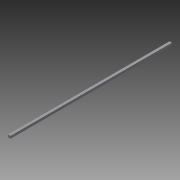
# Autodesk Inventor part: Standbein_aussen
Saved by Autodesk Inventor 2015 (Build 190159000, 159)
## iProperties
Created: 2018-03-07
Part Number: Standbein_aussen
Material: Generisch
Document SubType Name: Modeling
Designer: wepet
Density: 1 g/cm^3
Appearance: Vorgabe
Author: wepet
Autodesk Inventor part; units mm, degrees
ref_plane "YZ Plane" through (0, 0, 0) normal (1, 0, 0) x (0, 1, 0)
ref_plane "XZ Plane" through (0, 0, 0) normal (0, 1, 0) x (-1, 0, 0)
ref_plane "XY Plane" through (0, 0, 0) normal (0, 0, 1) x (1, 0, 0)
sketch "Skizze1" plane through (0, 0, 0) normal (0, 1, 0) x (-1, 0, 0)
  line L0 (15, 15) -> (-15, 15)
  line L1 (-15, 15) -> (-15, -15)
  line L2 (-15, -15) -> (15, -15)
  line L3 (15, -15) -> (15, 15)
  line L4 (0, 0) -> (15, 0) construction
  line L5 (0, 0) -> (0, -15) construction
  dimension "d0" = 30
  dimension "d1" = 30
  constraints: 12 end point, 2 horizontal, 2 midpoint, 2 parallel, 2 perpendicular
  measures "d0" distance of L2.end L0.start
  measures "d1" distance of L1.end L2.end
extrude "Extrusion1" add sketch "Skizze1" along normal blind 2000
sketch "Skizze2" plane through (15, 0, -15) normal (1, 0, 0) x (0, 0, -1)
  line L0 (-30, 0) -> (0, 0) projected
  line L1 (-15, 0) -> (-15, 50) construction
  dimension "d4" = 50
  constraints: 2 end point, 1 coincident, 1 vertical
  measures "d4" distance of L1.start L1.end
sketch "Skizze4" plane through (15, 0, 15) normal (0, 0, 1) x (1, 0, 0)
  line L0 (0, 50) -> (-30, 53.5507) construction
  line L1 (-30, 0) -> (-30, 53.5507) construction
  line L2 (-30, 0) -> (-30, 2000) construction
  line L3 (0, 0) -> (0, 2000) construction
  point P0 (-15, 0)
  dimension "d12" = 83.25
  constraints: 4 end point, 1 coincident, 1 point on line
  measures "d12" angle of L0 L3
sketch "Skizze5" plane through (-15, 0, 15) normal (-1, 0, 0) x (0, 0, 1)
  line L0 (0, 53.5507) -> (-30, 53.5507) construction
  line L1 (-30, 0) -> (-30, 2000) construction
  line L2 (-15, 0) -> (-15, 53.5507) construction
  constraints: 4 end point, 1 coincident, 1 horizontal, 1 midpoint, 1 point on line
hole "Bohrung2" at (15, 50, 0) direction (-0.9930685, 0.1175374, 0) diameter 10 end through all
delete faces "Fläche löschen1" heal yes whole lump no faces at (14.8701, 48.9025, 1.2475)
